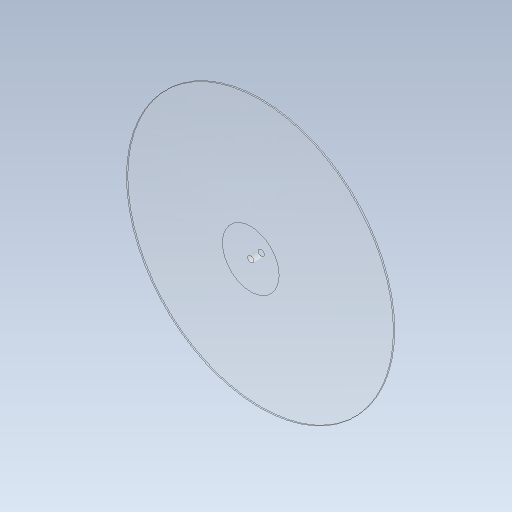
# Autodesk Inventor part: Props
Saved by Autodesk Inventor 2020 (Build 240168000, 168)
## iProperties
Part Number: Props
Material: GEDA Plexiglas
Document SubType Name: Modeling
Designer: Admin
Mass: 39.8365 g
Surface Area: 1026.57 cm^2
Volume: 248.978 cm^3
Density: 0.16 g/cm^3
Appearance: GEDA Plexiglas A
Gewicht: 0,040 kg
G_L: 0
G_H: 0
G_B: 0
InventorVersion: 2019.4
VAULT_Status: in Bearbeitung
Revision: -
Max. Breite: 0
Max. Höhe: 0
Max. Länge: 0
Max. Abmessungen: 0 x 0 x 0
Author: Admin
Autodesk Inventor part; units mm, degrees
note: some values were not read from the file. Left out: dimensions or parameters whose unit could not be read.
ref_plane "YZ Plane" through (0, 0, 0) normal (1, 0, 0) x (0, 1, 0)
ref_plane "XZ Plane" through (0, 0, 0) normal (0, 1, 0) x (-1, 0, 0)
ref_plane "XY Plane" through (0, 0, 0) normal (0, 0, 1) x (1, 0, 0)
sketch "Skizze1" plane through (0, 0, 0) normal (0, 1, 0) x (-1, 0, 0)
  circle A0 centre (0, 0) radius 3
  line L0 (-20, -4) -> (20, -4)
  line L1 (20, -4) -> (20, 4)
  line L2 (20, 4) -> (-20, 4)
  line L3 (-20, 4) -> (-20, -4)
  line L4 (-20, -4) -> (20, 4) construction
  line L5 (20, -4) -> (-20, 4) construction
  dimension "d0" = 6
  dimension "d1" = 40
  dimension "d2" = 8
  constraints: 12 end point, 2 midpoint, 2 parallel, 1 centre point, 1 coincident, 1 horizontal, 1 perpendicular
  measures "d0" diameter of A0
  measures "d1" distance of L2.end L1.end
  measures "d2" distance of L1.end L0.end
extrude "Extrusion1" add sketch "Skizze1" along normal blind 10
sketch "Skizze2" plane through (0, 0, 0) normal (0, 1, 0) x (-1, 0, 0)
  circle A0 centre (0, 0) radius 127
  circle A1 centre (0, 0) radius 3 projected
  dimension "d6" = 254
  constraints: 1 centre point, 1 concentric
  measures "d6" diameter of A0
extrude "Extrusion2" add sketch "Skizze2" along normal blind 10
chamfer "Fase1" distance 100 angle 5 1 edges at (127, 0, 0) measured on face at (84.8365, 0, -10.6241)
equation "\"G_L\" = 0"
equation "\"G_H\" = 0"
equation "\"G_B\" = 0"
